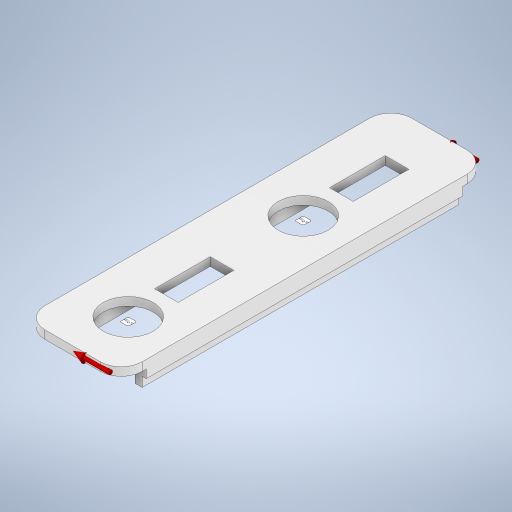
# Autodesk Inventor part: Soporte
Saved by Autodesk Inventor 2024.1 (Build 281209000, 209)
## iProperties
Created: 2023-07-29
Part Number: Soporte
Material: Plástico ABS
Document SubType Name: Modeling
Designer: Det-Pc
Density: 1.06 g/cm^3
Appearance: Suave - Blanco
Mass: 16.3095 g
Surface Area: 121.282 cm^2
Volume: 15.3863 cm^3
Author: Det-Pc
Autodesk Inventor part; units mm, degrees
ref_plane "YZ Plane" through (0, 0, 0) normal (1, 0, 0) x (0, 1, 0)
ref_plane "XZ Plane" through (0, 0, 0) normal (0, 1, 0) x (-1, 0, 0)
ref_plane "XY Plane" through (0, 0, 0) normal (0, 0, 1) x (1, 0, 0)
sketch "Boceto1" plane through (0, 0, 0) normal (0, 1, 0) x (-1, 0, 0)
  line L0 (10, 66) -> (-10, 66)
  line L1 (-17.5, 58.5) -> (-17.5, -58.5)
  line L2 (-10, -66) -> (10, -66)
  line L3 (17.5, -58.5) -> (17.5, 58.5)
  arc A0 (17.5, 58.5) -> (10, 66) centre (10, 58.5) ccw
  arc A1 (-10, 66) -> (-17.5, 58.5) centre (-10, 58.5) ccw
  arc A2 (-17.5, -58.5) -> (-10, -66) centre (-10, -58.5) ccw
  arc A3 (10, -66) -> (17.5, -58.5) centre (10, -58.5) ccw
  circle A4 centre (-1, 47) radius 9
  circle A5 centre (-1, -16) radius 9
  line L4 (3, 33.5) -> (-5.5, 33.5)
  line L5 (-5.5, 33.5) -> (-5.5, 13.5)
  line L6 (-5.5, 13.5) -> (3, 13.5)
  line L7 (3, 13.5) -> (3, 33.5)
  line L8 (3, -29.5) -> (-5.5, -29.5)
  line L9 (-5.5, -29.5) -> (-5.5, -49.5)
  line L10 (-5.5, -49.5) -> (3, -49.5)
  line L11 (3, -49.5) -> (3, -29.5)
  point P0 (0, 0)
  point P1 (17.5, 66)
  point P2 (-17.5, -66)
  point P3 (17.5, -66)
  point P4 (17.5, 0)
  point P5 (0, -66)
  point P6 (-1.25, 13.5)
  point P7 (-1.25, -49.5)
  point P8 (-1.25, 33.5)
  dimension "d0" = 35
  dimension "d1" = 132
  dimension "d2" = 7.5
  dimension "d5" = 8.5
  dimension "d8" = 20
  dimension "d9" = 12
  dimension "d10" = 43
  dimension "d11" = 16.5
  dimension "d12" = 13.5
  dimension "d13" = 16.5
  dimension "d15" = 18
  dimension "d16" = 13.5
  constraints: 24 end point, 8 point on circle, 8 tangent, 6 centre point, 6 parallel, 6 point on line, 5 midpoint, 4 equal radius, 3 horizontal, 3 perpendicular, 3 vertical alignment, 2 equal length, 1 horizontal alignment
  measures "d0" distance of point (-17.5, -66) point (17.5, -66)
  measures "d1" distance of point (17.5, -66) point (17.5, 66)
  measures "d2" radius of A0
  measures "d5" distance of L4.start L4.end
  measures "d8" distance of L10.end L8.start
  measures "d9" distance between parallel lines of L1 L9
  measures "d10" distance between parallel lines of L8 L6
  measures "d11" distance between parallel lines of L2 L10
  measures "d12" distance from line of L8 A5.centre
  measures "d13" distance from line of L1 A5.centre
  measures "d15" diameter of A4
  measures "d16" vertical distance of point (-1.25, 33.5) A4.centre
extrude "Extrusión1" add sketch "Boceto1" along normal blind 3
sketch "Boceto2" plane through (0, 0, 0) normal (0, -1, 0) x (1, 0, 0)
  line L0 (17.5, 57) -> (13.5, 57)
  line L1 (13.5, 57) -> (13.5, -57)
  line L2 (13.5, -57) -> (17.5, -57)
  line L3 (17.5, -57) -> (17.5, 57)
  line L4 (-10.5, 57) -> (-13, 57)
  line L5 (-13, 57) -> (-13, -57)
  line L6 (-13, -57) -> (-10.5, -57)
  line L7 (-10.5, -57) -> (-10.5, 57)
  line L8 (16, 57) -> (16, -57)
  line L9 (17.5, 58.5) -> (17.5, -58.5) projected
  point P0 (0, 0)
  point P1 (17.5, 0)
  point P2 (17.5, 0)
  point P3 (-10.5, 0)
  point P4 (13.5, 0)
  dimension "d19" = 4
  dimension "d20" = 114
  dimension "d21" = 2.5
  dimension "d22" = 2.5
  dimension "d23" = 24
  constraints: 18 end point, 5 parallel, 4 midpoint, 3 perpendicular, 2 horizontal, 2 horizontal alignment, 2 point on line, 1 coincident
  measures "d19" distance of L0.start L0.end
  measures "d20" distance of L2.end L0.start
  measures "d21" distance of L4.start L4.end
  measures "d22" distance between parallel lines of L1 L8
  measures "d23" distance between parallel lines of L1 L7
extrude "Extrusión2" add sketch "Boceto2" along normal blind 6.5 contours L8 L2 L1 L0 | L7 L6 L5 L4
extrude "Extrusión3" add sketch "Boceto2" along normal blind 3 contours L3 L2 L8 L0
